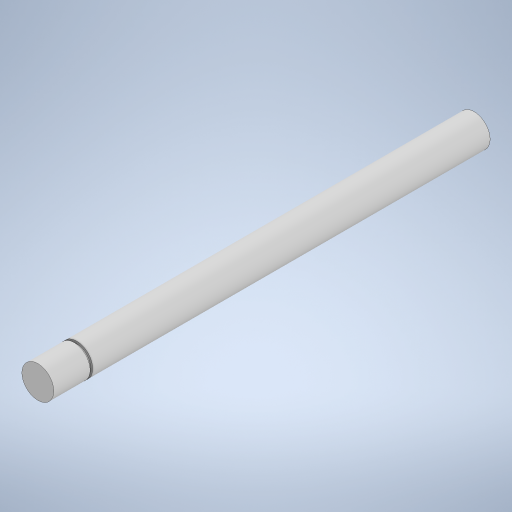
# Autodesk Inventor part: 3 Piston Rod
Saved by Autodesk Inventor 2024 (Build 280153000, 153)
## iProperties
Created: 2024-04-17
Part Number: 3 Piston Rod
Material: Generic
Document SubType Name: Modeling
Designer: Tommy Rohmann
Density: 1 g/cm^3
Appearance: Default
Author: Tommy Rohmann
Autodesk Inventor part; units mm, degrees
ref_plane "YZ Plane" through (0, 0, 0) normal (1, 0, 0) x (0, 1, 0)
ref_plane "XZ Plane" through (0, 0, 0) normal (0, 1, 0) x (-1, 0, 0)
ref_plane "XY Plane" through (0, 0, 0) normal (0, 0, 1) x (1, 0, 0)
sketch "Sketch1" plane through (0, 0, 0) normal (0, 1, 0) x (-1, 0, 0)
  line L0 (0, 0) -> (-11.1125, 0)
  line L1 (-11.1125, 0) -> (-11.1125, -334.6595)
  line L2 (-11.1125, -25.4) -> (-9.525, -25.4)
  line L3 (-9.525, -25.4) -> (-9.525, -27.178)
  line L4 (-9.525, -27.178) -> (-11.1125, -27.178)
  line L5 (0, 0) -> (0, -334.6595)
  line L6 (-11.1125, -304.8) -> (0, -304.8)
  dimension "d0" = 11.1125
  dimension "d2" = 334.6595
  dimension "d4" = 25.4
  dimension "d5" = 1.778
  dimension "d6" = 1.5875
  dimension "d7" = 304.8
  constraints: 14 end point, 4 point on line, 4 vertical, 3 perpendicular, 2 horizontal
  measures "d0" distance of point (0, 0) L0.end
  measures "d2" distance of L0.end L1.end
  measures "d4" distance between parallel lines of L0 L2
  measures "d5" distance between parallel lines of L4 L2
  measures "d6" distance between parallel lines of L1 L3
  measures "d7" distance between parallel lines of L0 L6
revolve "Revolution1" add sketch "Sketch1" angle 360 about axis through (0, 0, 0) along (0, 0, -1) contours L5 L6 L1 L4 L3 L2 L0
body "Solid1"
